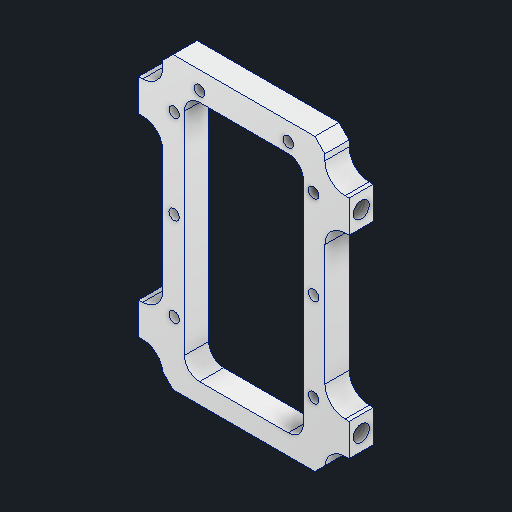
# Autodesk Inventor part: DynamixelServoMount
Saved by Autodesk Inventor 2025 (Build 290162000, 162)
## iProperties
Created: 2024-05-20
Part Number: DynamixelServoMount
Material: Aluminum 6061
Document SubType Name: Modeling
Designer: avsar
Density: 2.7 g/cm^3
Appearance: Aluminum - Flat
Author: avsar
Autodesk Inventor part; units mm, degrees
ref_plane "YZ Plane" through (0, 0, 0) normal (1, 0, 0) x (0, 1, 0)
ref_plane "XZ Plane" through (0, 0, 0) normal (0, 1, 0) x (-1, 0, 0)
ref_plane "XY Plane" through (0, 0, 0) normal (0, 0, 1) x (1, 0, 0)
sketch "Sketch1" plane through (0, 0, 0) normal (0, 0, 1) x (1, 0, 0)
  line L0 (-11, -29.75) -> (11, -29.75) construction
  line L1 (14.5, -26.25) -> (14.5, 26.25) construction
  line L2 (11, 29.75) -> (-11, 29.75) construction
  line L3 (-14.5, 26.25) -> (-14.5, -26.25) construction
  line L4 (-14.5, -29.75) -> (14.5, 29.75) construction
  line L5 (14.5, -29.75) -> (-14.5, 29.75) construction
  arc A0 (-11, 29.75) -> (-14.5, 26.25) centre (-11, 26.25) ccw construction
  arc A1 (14.5, 26.25) -> (11, 29.75) centre (11, 26.25) ccw construction
  arc A2 (11, -29.75) -> (14.5, -26.25) centre (11, -26.25) ccw
  arc A3 (-14.5, -26.25) -> (-11, -29.75) centre (-11, -26.25) ccw construction
  line L6 (-17.6, -35) -> (17.6, -35)
  line L7 (20.1, -32.5) -> (20.1, 34.5)
  line L8 (17.6, 37) -> (-17.6, 37)
  line L9 (-20.1, 34.5) -> (-20.1, -32.5)
  line L10 (-20.1, -35) -> (20.1, 37) construction
  line L11 (20.1, -35) -> (-20.1, 37) construction
  line L12 (-20.1, 34.5) -> (-17.6, 37)
  line L13 (-20.1, -32.5) -> (-17.6, -35)
  line L14 (17.6, -35) -> (20.1, -32.5)
  line L15 (17.6, 37) -> (20.1, 34.5)
  circle A4 centre (0, -15.25) radius 14 construction
  circle A5 centre (-17.3, -19.25) radius 1.3
  circle A6 centre (-17.3, 2.75) radius 1.3
  circle A7 centre (-17.3, 24.75) radius 1.3
  circle A8 centre (-11, 32.55) radius 1.3
  line L16 (0, -15.25) -> (0, -1.25) construction
  circle A9 centre (17.3, -19.25) radius 1.3
  circle A10 centre (17.3, 2.75) radius 1.3
  circle A11 centre (17.3, 24.75) radius 1.3
  circle A12 centre (11, 32.55) radius 1.3
  line L17 (-11, 30) -> (11, 30)
  arc A13 (14.75, 26.25) -> (11, 30) centre (11, 26.25) ccw
  line L18 (14.75, 26.25) -> (14.75, -26.25)
  arc A14 (11, -30) -> (14.75, -26.25) centre (11, -26.25) ccw
  line L19 (11, -30) -> (-11, -30)
  arc A15 (-14.75, -26.25) -> (-11, -30) centre (-11, -26.25) ccw
  line L20 (-14.75, -26.25) -> (-14.75, 26.25)
  arc A16 (-11, 30) -> (-14.75, 26.25) centre (-11, 26.25) ccw
  point P0 (0, 0)
  point P1 (0, 1)
  point P2 (0, 29.75)
  dimension "d14" = 28
  dimension "d0" = 29
  dimension "d1" = 59.5
  dimension "d2" = 3.5
  dimension "d3" = 40.2
  dimension "d4" = 72
  dimension "d6" = 2.5
  dimension "d7" = 2.5
  dimension "d8" = 2.5
  dimension "d9" = 2.5
  dimension "d10" = 2.5
  dimension "d11" = 2.5
  dimension "d12" = 2.5
  dimension "d13" = 2.5
  dimension "d15" = 45
  dimension "d16" = 2.6
  dimension "d17" = 17.3
  dimension "d18" = 4
  dimension "d19" = 2.6
  dimension "d20" = 22
  dimension "d21" = 2.6
  dimension "d22" = 22
  dimension "d24" = 2.6
  dimension "d26" = 7.8
  dimension "d27" = 11
  dimension "d28" = 1
  dimension "d51" = 0.25
  constraints: 42 end point, 16 centre point, 16 point on circle, 16 point on line, 8 tangent, 6 parallel, 5 midpoint, 5 vertical alignment, 4 symmetric about line, 3 equal radius, 3 perpendicular, 2 horizontal, 1 vertical, 13 other
  measures "d0" distance of L5.end L4.end
  measures "d1" distance of L4.end L5.start
  measures "d2" radius of A0
  measures "d3" distance of L11.end L10.end
  measures "d4" distance of L10.end L11.start
  measures "d6" distance of L9.start L11.end
  measures "d7" distance of L8.end L11.end
  measures "d8" distance of L9.end L10.start
  measures "d9" distance of L6.start L10.start
  measures "d10" distance of L6.end L11.start
  measures "d11" distance of L7.start L11.start
  measures "d12" distance of L8.start L10.end
  measures "d13" distance of L7.end L10.end
  measures "d15" distance from line of L2 L16.start
  measures "d16" diameter of A5
  measures "d17" horizontal distance of L16.start A5.centre
  measures "d18" vertical distance of L16.start A5.centre
  measures "d19" diameter of A6
  measures "d20" distance of A6.centre A5.centre
  measures "d21" diameter of A7
  measures "d22" distance of A6.centre A7.centre
  measures "d24" diameter of A8
  measures "d26" vertical distance of A7.centre A8.centre
  measures "d27" horizontal distance of point (0, 1) A8.centre
  measures "d28" distance of point (0, 0) point (0, 1)
  measures "d51" distance between parallel lines of L2 L17
extrude "Extrusion1" add sketch "Sketch1" along normal blind 6
sketch "Sketch2" plane through (0, 0, 6) normal (0, 0, 1) x (1, 0, 0)
  line L0 (26.1, 28) -> (26.1, 20)
  line L1 (20.1, -32.5) -> (20.1, 34.5) projected
  line L2 (26.1, 20) -> (20.1, 20)
  line L3 (26.1, 28) -> (20.1, 28)
  line L4 (-14.5, 0) -> (14.5, 0) construction
  line L5 (0, 29.4068) -> (0, -29.4068) construction
  line L6 (-26.1, 28) -> (-26.1, 20)
  line L7 (-26.1, 20) -> (-20.1, 20)
  line L8 (-26.1, 28) -> (-20.1, 28)
  line L9 (26.1, -28) -> (26.1, -20)
  line L10 (26.1, -20) -> (20.1, -20)
  line L11 (26.1, -28) -> (20.1, -28)
  line L12 (-26.1, -20) -> (-20.1, -20)
  line L13 (-26.1, -28) -> (-26.1, -20)
  line L14 (-26.1, -28) -> (-20.1, -28)
  line L15 (-20.1, 28) -> (-20.1, 20)
  line L16 (-20.1, 34.5) -> (-20.1, -32.5) projected
  line L17 (-20.1, -20) -> (-20.1, -28)
  line L18 (-20.1, 34.5) -> (-20.1, -32.5) projected
  point P0 (0, 0)
  point P1 (26.1, 24)
  point P2 (20.1, -20)
  point P3 (20.1, -28)
  point P4 (0, 0)
  dimension "d31" = 24
  dimension "d32" = 8
  dimension "d33" = 6
  constraints: 32 end point, 12 symmetric about line, 5 midpoint, 2 collinear, 2 perpendicular, 2 point on line, 1 vertical
  measures "d31" vertical distance of point (26.1, 24) point (0, 0)
  measures "d32" distance of L0.start L0.end
  measures "d33" distance of L0.start L3.end
extrude "Extrusion2" add sketch "Sketch2" against normal up to surface (6 mm away)
fillet "Fillet1" radius 5 8 edges at (20.1, 28, 3) (-20.1, 28, 3) (-20.1, -20, 3) (-20.1, -28, 3) (20.1, -28, 3) (20.1, 20, 3) (20.1, -20, 3) (-20.1, 20, 3)
sketch "Sketch3" plane through (-26.1, 20, 6) normal (-1, 0, 0) x (0, 0, 1)
  line L0 (-6, 0) -> (-6, 8) construction
  line L1 (0, 0) -> (-6, 0) construction
  line L2 (0, 8) -> (0, 0) construction
  line L3 (0, 8) -> (-6, 8) construction
  line L4 (0, 8) -> (-6, 0) construction
  circle A0 centre (-3, 4) radius 2
  line L5 (-6, -48) -> (-6, -40) construction
  line L6 (0, -48) -> (-6, -48) construction
  line L7 (0, -40) -> (0, -48) construction
  line L8 (0, -40) -> (-6, -40) construction
  line L9 (0, -40) -> (-6, -48) construction
  circle A1 centre (-3, -44) radius 2
  point P0 (-6, -20)
  dimension "d37" = 4
  dimension "d38" = 4
  constraints: 4 end point, 2 centre point, 2 midpoint
  measures "d37" diameter of A0
  measures "d38" diameter of A1
extrude "Extrusion3" cut sketch "Sketch3" against normal blind 6
mirror "Mirror1" about plane through (0, 0, 0) normal (1, 0, 0) of "Extrusion3"
thread "Thread1" size "M4x0.7" class "6H" standard "ANSI Metric M Profile" full length
thread "Thread2" size "M4x0.7" class "6H" standard "ANSI Metric M Profile" full length
thread "Thread3" size "M4x0.7" class "6H" standard "ANSI Metric M Profile" full length
thread "Thread4" size "M4x0.7" class "6H" standard "ANSI Metric M Profile" full length
equation "\"d7\" = d6"
equation "\"d8\" = d6"
equation "\"d9\" = d8"
equation "\"d10\" = d6"
equation "\"d11\" = d10"
equation "\"d12\" = d6"
equation "\"d13\" = d12"
body "Solid1"
